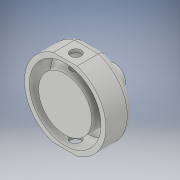
# Autodesk Inventor part: новая шайба потенциометра
Saved by Autodesk Inventor 2019.1 (Build 231200000, 200)
## iProperties
Created: 2018-08-27
Part Number: новая шайба потенциометра
Material: Типовые
Document SubType Name: Modeling
Designer: olege
Density: 1 g/cm^3
Appearance: По умолчанию
Author: olege
Autodesk Inventor part; units mm, degrees
ref_plane "YZ Plane" through (0, 0, 0) normal (1, 0, 0) x (0, 1, 0)
sketch "Эскиз1" plane through (0, 0, 0) normal (0, 0, 1) x (1, 0, 0)
  circle A0 centre (0, 0) radius 10.1
  circle A1 centre (0, 0) radius 11.5
  dimension "d0" = 20.2
  dimension "d1" = 23
  constraints: 2 centre point, 2 coincident
  measures "d0" diameter of A0
  measures "d1" diameter of A1
extrude "Выдавливание1" add sketch "Эскиз1" along normal blind 6
sketch "Эскиз2" plane through (0, 0, 0) normal (0, 0, -1) x (-1, 0, 0)
  circle A0 centre (0, 0) radius 11.5 projected
extrude "Выдавливание2" add sketch "Эскиз2" along normal blind 2
sketch "Эскиз3" plane through (0, 0, 0) normal (0, 1, 0) x (-1, 0, 0)
  circle A0 centre (0, 3) radius 1.5
  point P0 (0, 0)
  dimension "d6" = 3
  dimension "d7" = 3
  constraints: 1 centre point, 1 vertical alignment
  measures "d6" diameter of A0
  measures "d7" distance of point (0, 0) A0.centre
extrude "Выдавливание3" cut sketch "Эскиз3" along normal mid plane 36.925
ref_plane "РабПлоскость1" through (0, -11.5, 0) normal (0, 1, 0) x (-1, 0, 0)
sketch "Эскиз5" plane through (0, -11.5, 0) normal (0, 1, 0) x (-1, 0, 0)
  circle A0 centre (1.2165, -4.866) radius 25.5876
  point P0 (0, 0)
  constraints: 1 centre point
extrude "Выдавливание4" cut sketch "Эскиз5" along normal blind 0.5
ref_plane "РабПлоскость2" through (0, 11.5, 0) normal (0, 1, 0) x (-1, 0, 0)
sketch "Эскиз6" plane through (0, 11.5, 0) normal (0, 1, 0) x (-1, 0, 0)
  circle A0 centre (5.3505, 13.4629) radius 49.845
  point P0 (0, 0)
  constraints: 1 centre point
extrude "Выдавливание5" cut sketch "Эскиз6" against normal blind 0.5
sketch "Эскиз7" plane through (0, 0, -2) normal (0, 0, -1) x (-1, 0, 0)
  circle A0 centre (0, 0) radius 3
  line L0 (1.4491, -1.15) -> (-1.4491, -1.15)
  line L1 (-1.4491, 1.15) -> (1.4491, 1.15)
  line L2 (2.2473, -1.15) -> (-2.2473, 1.15) construction
  line L3 (-2.2473, -1.15) -> (2.2473, 1.15) construction
  arc A1 (-1.4491, 1.15) -> (-1.4491, -1.15) centre (0, 0) ccw
  arc A2 (1.4491, -1.15) -> (1.4491, 1.15) centre (0, 0) ccw
  line L4 (-1.5875, -1.45) -> (1.5875, -1.45)
  arc A3 (1.5875, -1.45) -> (1.5875, 1.45) centre (0, 0) ccw
  line L5 (1.5875, 1.45) -> (-1.5875, 1.45)
  arc A4 (-1.5875, 1.45) -> (-1.5875, -1.45) centre (0, 0) ccw
  dimension "d16" = 6
  dimension "d18" = 2.3
  dimension "d19" = 1.85
  dimension "d20" = 1.85
  dimension "d21" = 2.3
  dimension "d22" = 1.15
  dimension "d27" = 0.3
  constraints: 12 end point, 8 point on circle, 5 centre point, 2 coincident, 2 midpoint, 2 parallel, 1 horizontal, 3 other
  measures "d16" diameter of A0
  measures "d18" distance of L3.start L2.end
  measures "d19" radius of A2
  measures "d20" radius of A1
  measures "d21" distance between parallel lines of L0 L1
  measures "d22" distance from line of L0 point (0, 0)
  measures "d27" distance between parallel lines of L0 L4
fillet "Сопряжение2" radius 2 4 edges at (11.5, 0, -2) (-11.5, 0, -2) (0, -11, -2) (0, 11, -2)
sketch "Эскиз8" plane through (0, 0, 0) normal (0, 0, 1) x (1, 0, 0)
  circle A0 centre (0, 0) radius 7.5
  dimension "d31" = 15
  constraints: 1 centre point, 1 coincident
  measures "d31" diameter of A0
extrude "Выдавливание8" add sketch "Эскиз7" along normal blind 6 contours A0
extrude "Выдавливание9" add sketch "Эскиз8" along normal blind 6
fillet "Сопряжение4" radius 3 1 edges at (3, 0, -2)
sketch "Эскиз9" plane through (0, 11, 0) normal (0, 1, 0) x (1, 0, 0)
  circle A0 centre (0, -3) radius 1.5 projected
  point P0 (0, 0)
extrude "Выдавливание10" cut sketch "Эскиз9" against normal blind 31.275
